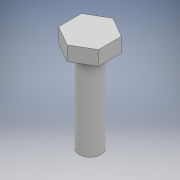
# Autodesk Inventor part: Tornillo para Motor Pololu
Saved by Autodesk Inventor 2018.3 (Build 223284000, 284)
## iProperties
Created: 2021-02-19
Part Number: Tornillo para Motor Pololu
Material: Genérico
Document SubType Name: Modeling
Designer: SERGIO ROMO
Density: 1 g/cm^3
Appearance: Valor por defecto
Author: SERGIO ROMO
Autodesk Inventor part; units mm, degrees
ref_plane "YZ Plane" through (0, 0, 0) normal (1, 0, 0) x (0, 1, 0)
ref_plane "XZ Plane" through (0, 0, 0) normal (0, 1, 0) x (-1, 0, 0)
ref_plane "XY Plane" through (0, 0, 0) normal (0, 0, 1) x (1, 0, 0)
sketch "Boceto1" plane through (0, 0, 0) normal (0, 0, 1) x (1, 0, 0)
  line L0 (-2.75, 1.5839) -> (-0.0033, 3.1735)
  line L1 (-0.0033, 3.1735) -> (2.7467, 1.5896)
  line L2 (2.7467, 1.5896) -> (2.75, -1.5839)
  line L3 (2.75, -1.5839) -> (0.0033, -3.1735)
  line L4 (0.0033, -3.1735) -> (-2.7467, -1.5896)
  line L5 (-2.7467, -1.5896) -> (-2.75, 1.5839)
  point P0 (0, 0)
  point P1 (0, 0)
  constraints: 12 end point, 13 other
extrude "Extrusión1" add sketch "Boceto1" against normal blind 2
sketch "Boceto2" plane through (0, 0, -2) normal (0, 0, -1) x (-1, 0, 0)
  circle A0 centre (0, 0) radius 1.5
  dimension "d3" = 3
  constraints: 1 centre point, 1 coincident
  measures "d3" diameter of A0
extrude "Extrusión2" add sketch "Boceto2" along normal blind 12
